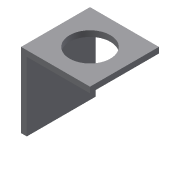
# Autodesk Inventor part: motorbracket
Saved by Autodesk Inventor 2015 (Build 190159000, 159)
## iProperties
Created: 2015-03-13
Part Number: motorbracket
Material: Generic
Document SubType Name: Modeling
Designer: Jaden
Density: 1 g/cm^3
Appearance: Default
Author: Jaden
Autodesk Inventor part; units mm, degrees
ref_plane "YZ Plane" through (0, 0, 0) normal (1, 0, 0) x (0, 1, 0)
ref_plane "XZ Plane" through (0, 0, 0) normal (0, 1, 0) x (-1, 0, 0)
ref_plane "XY Plane" through (0, 0, 0) normal (0, 0, 1) x (1, 0, 0)
sketch "Sketch1" plane through (0, 0, 0) normal (0, 0, 1) x (1, 0, 0)
  line L0 (0, 0) -> (6.35, 0)
  line L1 (6.35, 0) -> (6.35, 76.2)
  line L2 (6.35, 76.2) -> (76.2, 76.2)
  line L3 (76.2, 76.2) -> (76.2, 82.55)
  line L4 (76.2, 82.55) -> (0, 82.55)
  line L5 (0, 82.55) -> (0, 0)
  dimension "d0" = 6.35
  dimension "d1" = 76.2
  dimension "d2" = 90
  dimension "d3" = 69.85
  dimension "d4" = 6.35
  constraints: 12 end point, 5 perpendicular, 1 horizontal
  measures "d0" distance of L0.start L0.end
  measures "d1" distance of L0.end L1.end
  measures "d2" angle of L1 L0
  measures "d3" distance of L1.end L2.end
  measures "d4" distance of L2.end L3.end
extrude "Extrusion1" add sketch "Sketch1" along normal blind 76.2
hole "Hole1" at (38.1, 82.55, 38.1) direction (0, -1, 0) diameter 45.0088 end through all
body "Solid1"
